Autodesk Inventor part; units mm, degrees
(part 3 of 3)
sketch "Sketch6" plane through (0, 0, 0) normal (1, 0, 0) x (0, 1, 0)
  line L0 (31.6549, 6.0594) -> (32.075, 5.6953)
  line L1 (32.075, 5.6953) -> (32.3975, 6.0674)
  line L2 (32.3975, 6.0674) -> (31.9774, 6.4315)
  line L3 (31.9774, 6.4315) -> (31.6549, 6.0594)
  line L4 (31.4402, 6.2454) -> (31.0322, 6.5991)
  line L5 (31.0322, 6.5991) -> (31.3547, 6.9712)
  line L6 (31.3547, 6.9712) -> (31.7627, 6.6176)
  line L7 (31.7627, 6.6176) -> (31.4402, 6.2454)
  line L8 (30.8068, 6.7944) -> (30.4919, 7.0673)
  line L9 (30.4919, 7.0673) -> (30.8634, 7.4959)
  line L10 (30.8634, 7.4959) -> (31.1783, 7.223)
  line L11 (31.1783, 7.223) -> (30.8068, 6.7944)
  line L12 (30.3122, 7.223) -> (29.8518, 7.6221)
  line L13 (29.8518, 7.6221) -> (30.2652, 8.099)
  line L14 (30.2652, 8.099) -> (30.7256, 7.7)
  line L15 (30.7256, 7.7) -> (30.3122, 7.223)
  line L16 (29.6591, 7.789) -> (29.2369, 8.328)
  line L17 (29.2369, 8.328) -> (29.9785, 8.9091)
  line L18 (29.9785, 8.9091) -> (30.4008, 8.3701)
  line L19 (30.4008, 8.3701) -> (29.6591, 7.789)
  line L20 (29.0128, 8.5054) -> (28.2357, 9.8579)
  line L21 (28.2357, 9.8579) -> (29.2002, 10.4121)
  line L22 (29.2002, 10.4121) -> (29.9773, 9.0596)
  line L23 (29.9773, 9.0596) -> (29.0128, 8.5054)
  line L24 (28.1313, 10.0396) -> (27.6871, 11.5769)
  line L25 (27.6871, 11.5769) -> (29.0097, 11.9591)
  line L26 (29.0097, 11.9591) -> (29.4539, 10.4217)
  line L27 (29.4539, 10.4217) -> (28.1313, 10.0396)
  line L28 (27.6048, 11.8616) -> (27.451, 13.6632)
  line L29 (27.451, 13.6632) -> (28.7507, 13.7742)
  line L30 (28.7507, 13.7742) -> (28.9045, 11.9726)
  line L31 (28.9045, 11.9726) -> (27.6048, 11.8616)
  line L32 (27.431, 13.8981) -> (27.5279, 15.4838)
  line L33 (27.5279, 15.4838) -> (29.2753, 15.3769)
  line L34 (29.2753, 15.3769) -> (29.1783, 13.7913)
  line L35 (29.1783, 13.7913) -> (27.431, 13.8981)
  line L36 (27.5433, 15.735) -> (27.7311, 16.384)
  line L37 (27.7311, 16.384) -> (29.5449, 15.8591)
  line L38 (29.5449, 15.8591) -> (29.3571, 15.21)
  line L39 (29.3571, 15.21) -> (27.5433, 15.735)
  point P0 (0, 0)
  constraints: 80 end point, 20 parallel, 12 point on line, 10 perpendicular
sketch "Sketch5" plane through (11.5, 25.5, 11.5) normal (0.5, 0.7071, -0.5) x (-0.7071, 0, -0.7071)
  line L0 (6.8252, -1.4428) -> (7.8817, -1.4428)
  line L1 (7.8817, -1.4428) -> (7.8817, -0.2694)
  line L2 (7.8817, -0.2694) -> (6.8252, -0.2694)
  line L3 (6.8252, -0.2694) -> (6.8252, -1.4428)
  line L4 (7.7834, -0.0942) -> (7.8817, 1.0177)
  line L5 (7.8817, 1.0177) -> (6.8531, 1.1086)
  line L6 (6.8531, 1.1086) -> (6.7549, -0.0033)
  line L7 (6.7549, -0.0033) -> (7.7834, -0.0942)
  line L8 (7.9744, 1.3229) -> (8.1838, 2.5507)
  line L9 (8.1838, 2.5507) -> (6.9188, 2.7665)
  line L10 (6.9188, 2.7665) -> (6.7094, 1.5387)
  line L11 (6.7094, 1.5387) -> (7.9744, 1.3229)
  line L12 (8.2323, 2.835) -> (8.6796, 3.9697)
  line L13 (8.6796, 3.9697) -> (7.2053, 4.5509)
  line L14 (7.2053, 4.5509) -> (6.758, 3.4162)
  line L15 (6.758, 3.4162) -> (8.2323, 2.835)
  line L16 (8.7942, 4.2603) -> (9.2218, 4.9952)
  line L17 (9.2218, 4.9952) -> (8.0469, 5.6787)
  line L18 (8.0469, 5.6787) -> (7.6193, 4.9438)
  line L19 (7.6193, 4.9438) -> (8.7942, 4.2603)
  line L20 (9.4056, 5.3112) -> (10.1998, 6.1602)
  line L21 (10.1998, 6.1602) -> (9.3216, 6.9817)
  line L22 (9.3216, 6.9817) -> (8.5274, 6.1328)
  line L23 (8.5274, 6.1328) -> (9.4056, 5.3112)
  line L24 (10.5561, 6.3427) -> (11.3524, 6.8618)
  line L25 (11.3524, 6.8618) -> (10.667, 7.9132)
  line L26 (10.667, 7.9132) -> (9.8707, 7.3941)
  line L27 (9.8707, 7.3941) -> (10.5561, 6.3427)
  line L28 (11.6904, 7.0821) -> (12.8584, 7.6536)
  line L29 (12.8584, 7.6536) -> (12.0601, 9.2853)
  line L30 (12.0601, 9.2853) -> (10.892, 8.7138)
  line L31 (10.892, 8.7138) -> (11.6904, 7.0821)
  line L32 (13.0567, 7.7507) -> (14.3838, 8.2969)
  line L33 (14.3838, 8.2969) -> (13.7539, 9.8271)
  line L34 (13.7539, 9.8271) -> (12.4269, 9.2809)
  line L35 (12.4269, 9.2809) -> (13.0567, 7.7507)
  line L36 (14.6205, 8.5158) -> (15.5759, 8.6325)
  line L37 (15.5759, 8.6325) -> (15.4151, 9.9488)
  line L38 (15.4151, 9.9488) -> (14.4597, 9.8321)
  line L39 (14.4597, 9.8321) -> (14.6205, 8.5158)
  point P0 (16.2635, -18.0312)
  constraints: 80 end point, 20 parallel, 10 perpendicular, 6 point on line, 1 horizontal
body "Solid1"
